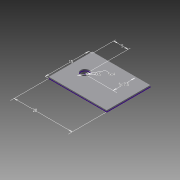
# Autodesk Inventor part: SzigeteloAlatetTranzisztor
Saved by Autodesk Inventor 2015 SP1 (Build 190203100, 203)
## iProperties
Created: 2014-10-30
Part Number: SzigeteloAlatetTranzisztor
Material: Generic
Document SubType Name: Modeling
Designer: laca
Density: 1 g/cm^3
Appearance: Default
Mass: 0.162959 g
Surface Area: 6.91549 cm^2
Volume: 0.162959 cm^3
Author: laca
Autodesk Inventor part; units mm, degrees
ref_plane "YZ Plane" through (0, 0, 0) normal (1, 0, 0) x (0, 1, 0)
ref_plane "XZ Plane" through (0, 0, 0) normal (0, 1, 0) x (-1, 0, 0)
ref_plane "XY Plane" through (0, 0, 0) normal (0, 0, 1) x (1, 0, 0)
sketch "Sketch1" plane through (0, 0, 0) normal (0, 1, 0) x (-1, 0, 0)
  line L0 (20, 15) -> (0, 15)
  line L1 (0, 15) -> (0, 0)
  line L2 (0, 0) -> (20, 0)
  line L3 (20, 0) -> (20, 15)
  circle A0 centre (15, 7.5) radius 1.5
  circle A1 centre (15, 7.5) radius 2
  dimension "d0" = 15
  dimension "d1" = 20
  dimension "d2" = 7.5
  dimension "d3" = 5
  dimension "d5" = 0.5
  dimension "d14" = 4
  constraints: 8 end point, 2 centre point, 2 parallel, 1 coincident, 1 horizontal, 1 perpendicular
  measures "d0" distance of L2.end L0.start
  measures "d1" distance of L0.start L0.end
  measures "d2" distance from line of L2 A0.centre
  measures "d3" distance from line of L3 A0.centre
  measures "d5" radial gap between concentric circles of A1 A0
  measures "d14" diameter of A1
extrude "Extrusion1" add sketch "Sketch1" along normal blind 0.5 contours L3 L2 L1 L0 | A1
extrude "Extrusion2" add sketch "Sketch1" against normal blind 3 contours A1
equation "\"d2\" = 0.5 * d0"
equation "\"d14\" = TranzisztoJukAtmero"
equation "\"TranzisztoJukAtmero\" = 4"
body "Solid1"
